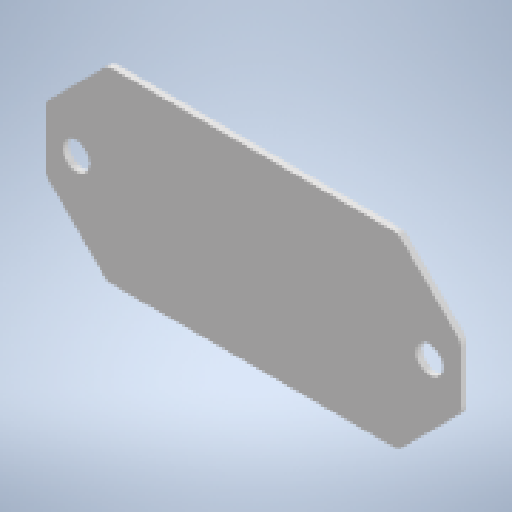
# Autodesk Inventor part: MSC 128 base plate
Saved by Autodesk Inventor 2025 (Build 290162010, 162A)
## iProperties
Created: 2024-07-01
Part Number: MSC 128 base plate
Material: Stainless Steel
Document SubType Name: Sheet Metal
Designer: admin
Density: 8 g/cm^3
Sheet Metal Rule: AISI304 2mm Die16
Appearance: Default
Author: pokla
Autodesk Inventor part; units mm, degrees
ref_plane "YZ Plane" through (0, 0, 0) normal (1, 0, 0) x (0, 1, 0)
ref_plane "XZ Plane" through (0, 0, 0) normal (0, 1, 0) x (-1, 0, 0)
ref_plane "XY Plane" through (0, 0, 0) normal (0, 0, 1) x (1, 0, 0)
sketch "Sketch1" plane through (0, 0, 0) normal (0, 1, 0) x (-1, 0, 0)
  line L0 (40, 40) -> (-40, 40) construction
  line L1 (-40, 40) -> (-40, -40) construction
  line L2 (-40, -40) -> (40, -40) construction
  line L3 (40, -40) -> (40, 40) construction
  line L4 (-40, 40) -> (40, -40) construction
  line L5 (100, -45) -> (-100, -45)
  line L6 (-100, -45) -> (-100, 45)
  line L7 (-100, 45) -> (100, 45)
  line L8 (100, 45) -> (100, -45)
  circle A0 centre (85, 0) radius 6.5
  circle A1 centre (-85, 0) radius 6.5
  line L9 (0, 40) -> (0, -40) construction
  line L10 (100, 15) -> (70, 45)
  line L11 (-70, 45) -> (-100, 15)
  line L12 (100, -15) -> (70, -45)
  line L13 (-100, -15) -> (-70, -45)
  line L14 (0, 0) -> (-40, 0) construction
  point P0 (0, 0)
  point P1 (0, 0)
  dimension "d2" = 80
  dimension "d3" = 80
  dimension "d17" = 5
  dimension "d20" = 45
  dimension "d23" = 15
  dimension "d24" = 30
  dimension "d26" = 45
  dimension "d27" = 13
  measures "d2" distance of L2.end L1.end
  measures "d3" distance of L1.end L0.end
  measures "d17" distance between parallel lines of L5 L2
  measures "d20" distance from line of L1 A1.centre
  measures "d23" distance from line of L6 A1.centre
  measures "d24" distance of L13.start L11.end
  measures "d26" angle of L6 L11
  measures "d27" diameter of A0
extrude "Plate1" add sketch "Sketch1" along normal blind 3 contours L5 L13 L6 L11 L7 L10 L8 L12
fillet "Corner Round2" radius 6 8 edges at (-70, 1.5, 45) (70, 1.5, 45) (100, 1.5, 15) (100, 1.5, -15) (70, 1.5, -45) (-100, 1.5, 15) (-100, 1.5, -15) (-70, 1.5, -45)
equation "\"d20\" = d19"
equation "\"d23\" = d22"
equation "\"BendReliefWidth\" = Thickness"
equation "\"BendReliefDepth\" = 0.5 * Thickness"
equation "\"CornerReliefSize\" = 4 * Thickness"
equation "\"MinimumRemnant\" = 2 * Thickness"
equation "\"TransitionRadius\" = BendRadius"
equation "\"JacobiRadiusSize\" = BendRadius"
equation "\"GapSize\" = Thickness"
equation "\"d19\" = 45"
equation "\"d22\" = 15"
body "Solid1"
